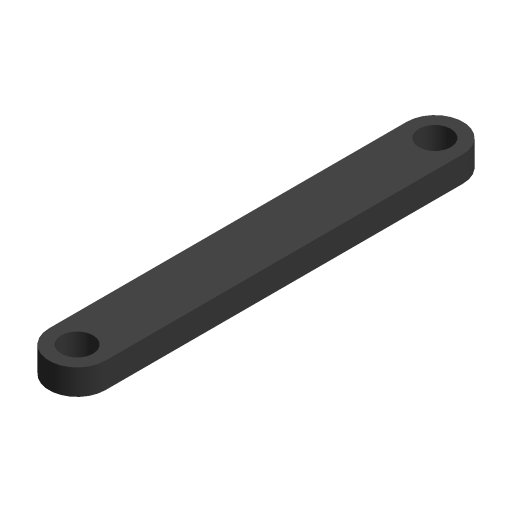
# Autodesk Inventor part: Camera retention
Saved by Autodesk Inventor 2024 (Build 280153000, 153)
## iProperties
Part Number: Camera retention
Material: Generic
Document SubType Name: Modeling
Designer: Jamie
Appearance: Default
Author: Jamie
Autodesk Inventor part; units mm, degrees
ref_plane "YZ Plane" through (0, 0, 0) normal (1, 0, 0) x (0, 1, 0)
ref_plane "XZ Plane" through (0, 0, 0) normal (0, 1, 0) x (-1, 0, 0)
ref_plane "XY Plane" through (0, 0, 0) normal (0, 0, 1) x (1, 0, 0)
sketch "Sketch1" plane through (0, 0, 0) normal (0, 1, 0) x (-1, 0, 0)
  line L0 (0, 0) -> (0, -28)
  circle A0 centre (2.2, 0) radius 1.25
  circle A1 centre (2.2, -28) radius 1.25
  arc A2 (4.4, 0) -> (0, 0) centre (2.2, 0) ccw
  arc A3 (0, -28) -> (4.4, -28) centre (2.2, -28) ccw
  line L1 (4.4, 0) -> (4.4, -28)
  dimension "d0" = 28
  dimension "d1" = 2.5
  dimension "d2" = 2.5
  dimension "d3" = 2.2
  dimension "d4" = 2.2
  constraints: 4 centre point, 4 end point, 4 point on circle, 2 coincident, 2 tangent, 1 vertical
  measures "d0" distance of L0.start L0.end
  measures "d1" diameter of A0
  measures "d2" diameter of A1
  measures "d3" distance of L0.start A0.centre
  measures "d4" distance of L0.end A1.centre
extrude "Extrusion1" add sketch "Sketch1" along normal blind 2
body "Solid1"
